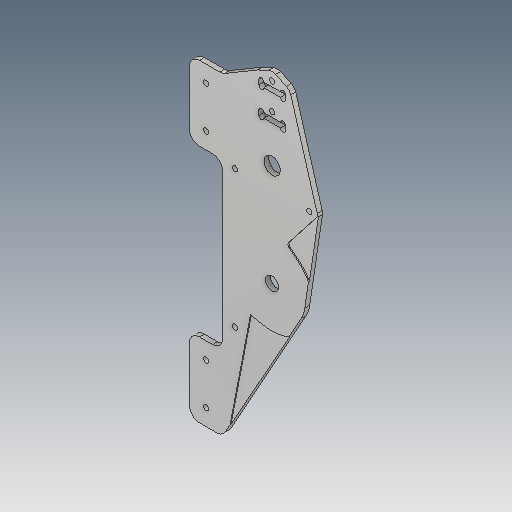
# Autodesk Inventor part: Pitch_B
Saved by Autodesk Inventor 2019.4 (Build 234330000, 330)
## iProperties
Created: 2019-06-11
Part Number: Pitch_B
Material: アルミニウム
Document SubType Name: Modeling
Designer: AzLIer
Density: 2.7 g/cm^3
Appearance: アルミニウム - つや出し
Mass: 74.3393 g
Surface Area: 210.238 cm^2
Volume: 27.5331 cm^3
Author: AzLIer
Autodesk Inventor part; units mm, degrees
ref_plane "YZ Plane" through (0, 0, 0) normal (1, 0, 0) x (0, 1, 0)
ref_plane "XZ Plane" through (0, 0, 0) normal (0, 1, 0) x (-1, 0, 0)
ref_plane "XY Plane" through (0, 0, 0) normal (0, 0, 1) x (1, 0, 0)
sketch "スケッチ1" plane through (0, 0, 0) normal (0, 0, 1) x (1, 0, 0)
  arc A0 (0, -120) -> (0, 120) centre (0, 0) ccw
  line L0 (0, 120) -> (0, -120)
  dimension "d0" = 120
  constraints: 2 end point, 2 point on circle, 1 centre point, 1 coincident, 1 vertical
  measures "d0" radius of A0
extrude "押し出し1" add sketch "スケッチ1" along normal blind 3
sketch "スケッチ2" plane through (0, 0, 0) normal (0, 0, -1) x (-1, 0, 0)
  line L0 (0, 120) -> (0, -120) projected
  line L1 (0, 120) -> (50, 120)
  line L2 (50, 120) -> (50, -120)
  line L3 (50, -120) -> (0, -120)
  line L4 (0, -120) -> (0, 120)
  point P0 (0, 0)
  dimension "d3" = 50
  constraints: 8 end point, 2 parallel, 1 horizontal, 1 perpendicular, 1 point on line
  measures "d3" distance of L0.start L1.end
extrude "押し出し2" add sketch "スケッチ2" against normal blind 3
sketch "スケッチ3" plane through (0, 0, 3) normal (0, 0, 1) x (1, 0, 0)
  line L0 (-50, 120) -> (-50, -120) projected
  line L1 (-50, 40) -> (-40, 40)
  line L2 (-40, 40) -> (-40, -40)
  line L3 (-40, -40) -> (-50, -40)
  line L4 (-50, -40) -> (-50, 40)
  line L5 (-40, 60) -> (-40, -60) construction
  circle A0 centre (-40, 60) radius 1.6
  circle A1 centre (-40, -60) radius 1.6
  point P0 (0, 0)
  point P1 (-50, 0)
  point P2 (-40, 0)
  point P3 (-40, 0)
  dimension "d8" = 10
  dimension "d9" = 80
  dimension "d10" = 120
  dimension "d11" = 10
  dimension "d12" = 3.2
  dimension "d13" = 3.2
  constraints: 10 end point, 4 midpoint, 3 coincident, 2 centre point, 2 parallel, 1 horizontal, 1 perpendicular, 1 vertical
  measures "d8" distance of L2.end L3.end
  measures "d9" distance of L1.end L2.end
  measures "d10" distance of L5.start L5.end
  measures "d11" distance between parallel lines of L0 L5
  measures "d12" diameter of A0
  measures "d13" diameter of A1
extrude "押し出し3" cut sketch "スケッチ3" against normal through all
sketch "スケッチ4" plane through (0, 0, 3) normal (0, 0, 1) x (1, 0, 0)
  circle A0 centre (0, 0) radius 4
  dimension "d14" = 8
  constraints: 1 centre point, 1 coincident
  measures "d14" diameter of A0
extrude "押し出し4" cut sketch "スケッチ4" against normal blind 3
sketch "スケッチ5" plane through (0, 0, 3) normal (0, 0, 1) x (1, 0, 0)
  circle A0 centre (0, 61.8122) radius 3 projected
  circle A1 centre (0, 61.8122) radius 5
  point P0 (0, 0)
  dimension "d17" = 10
  constraints: 1 centre point, 1 coincident
  measures "d17" diameter of A1
extrude "押し出し5" cut sketch "スケッチ5" against normal blind 3 contours A0 | A1
sketch "スケッチ7" plane through (0, 0, 3) normal (0, 0, 1) x (1, 0, 0)
  line L0 (15.7, 89.1122) -> (-15.7, 89.1122) projected
  line L1 (8, 87.1122) -> (-8, 87.1122)
  line L2 (-8, 87.1122) -> (-8, 84.1122)
  line L3 (-8, 84.1122) -> (8, 84.1122)
  line L4 (8, 84.1122) -> (8, 87.1122)
  arc A0 (-8, 84.1122) -> (-5, 84.1122) centre (-6.5, 84.1122) ccw
  arc A1 (5, 84.1122) -> (8, 84.1122) centre (6.5, 84.1122) ccw
  arc A2 (8, 87.1122) -> (5, 87.1122) centre (6.5, 87.1122) ccw
  arc A3 (-5, 87.1122) -> (-8, 87.1122) centre (-6.5, 87.1122) ccw
  circle A4 centre (0, 90.1122) radius 1.6
  point P0 (0, 0)
  point P1 (0, 87.1122)
  point P2 (0, 89.1122)
  dimension "d20" = 2
  dimension "d21" = 16
  dimension "d22" = 3
  dimension "d23" = 1.5
  dimension "d26" = 3.2
  dimension "d27" = 3
  constraints: 8 end point, 8 point on circle, 8 point on line, 5 centre point, 3 equal radius, 2 midpoint, 2 parallel, 2 vertical alignment, 1 horizontal, 1 perpendicular
  measures "d20" distance between parallel lines of L0 L1
  measures "d21" distance of L2.end L3.end
  measures "d22" distance of L3.end L1.start
  measures "d23" radius of A2
  measures "d26" diameter of A4
  measures "d27" distance of point (0, 87.112) A4.centre
extrude "押し出し6" cut sketch "スケッチ7" against normal blind 3
pattern_linear "矩形状パターン1" count 2 spacing 16 along (0, 1, 0) of "押し出し6"
sketch "スケッチ9" plane through (0, 0, 3) normal (0, 0, 1) x (1, 0, 0)
  circle A0 centre (0, 61.8122) radius 4 construction
  circle A1 centre (0, 0) radius 4 construction
  circle A2 centre (22.5, 49) radius 1.6 projected
  circle A3 centre (-22.5, -34) radius 1.6 projected
  circle A4 centre (-22.5, 49) radius 1.6 projected
  line L0 (25.0237, 50.6221) -> (12.6183, 69.9225) construction
  arc A5 (12.6183, 69.9225) -> (-12.6183, 69.9226) centre (0, 61.8122) ccw construction
  line L1 (-12.6183, 69.9226) -> (-25.0237, 50.6221) construction
  arc A6 (-25.0237, 50.6221) -> (-25.5, 49) centre (-22.5, 49) ccw construction
  line L2 (-25.5, 49) -> (-25.5, -34) construction
  arc A7 (-25.5, -34) -> (-20.5963, -36.3186) centre (-22.5, -34) ccw construction
  line L3 (-20.5963, -36.3186) -> (9.5184, -11.5931) construction
  arc A8 (9.5184, -11.5931) -> (14.6828, -3.0686) centre (0, 0) ccw construction
  line L4 (14.6828, -3.0686) -> (25.4366, 48.3863) construction
  arc A9 (25.4366, 48.3863) -> (25.0237, 50.6221) centre (22.5, 49) ccw construction
  point P0 (0, 0)
extrude "押し出し8" cut sketch "スケッチ9" against normal blind 3
sketch "スケッチ8" plane through (0, 0, 3) normal (0, 0, 1) x (1, 0, 0)
  arc A0 (17.4743, -9.7287) -> (19.7797, -2.9601) centre (0, 0) ccw
  line L0 (17.4743, -9.7287) -> (-30, -95)
  circle A1 centre (22.5, 49) radius 1.6 projected
  circle A2 centre (-22.5, 49) radius 1.6 projected
  circle A3 centre (-22.5, -34) radius 1.6 projected
  arc A4 (27.4449, 48.26) -> (27.2948, 50.4177) centre (22.5, 49) ccw
  line L1 (27.4449, 48.26) -> (19.7797, -2.9601)
  arc A5 (11.2948, 104.5299) -> (8.5953, 107.652) centre (6.5, 103.1122) ccw
  arc A6 (2.0953, 110.652) -> (-2.0953, 110.652) centre (0, 106.1122) ccw
  line L2 (8.5953, 107.652) -> (2.0953, 110.652)
  line L3 (27.2948, 50.4177) -> (11.2948, 104.5299)
  line L4 (-2.0953, 110.652) -> (-8.5953, 107.652)
  arc A7 (-8.5953, 107.652) -> (-9.0487, 107.4138) centre (-6.5, 103.1122) ccw
  line L5 (-9.0487, 107.4138) -> (-30, 95)
  circle A8 centre (-40, 85) radius 1.6 projected
  line L6 (-50, 50) -> (-30, 50) projected
  line L7 (-30, 95) -> (-30, 50) projected
  line L8 (-50, 95) -> (-30, 95) projected
  line L9 (-50, 50) -> (-50, 95) projected
  circle A9 centre (-40, 60) radius 1.6 projected
  circle A10 centre (-40, -85) radius 1.6 projected
  circle A11 centre (-40, -60) radius 1.6 projected
  line L10 (-30, -50) -> (-50, -50) projected
  line L11 (-50, -95) -> (-50, -50) projected
  line L12 (-30, -95) -> (-50, -95) projected
  line L13 (-30, -50) -> (-30, -95) projected
  line L14 (-30, 50) -> (-30, -50)
  point P0 (-47, -55)
  point P1 (-50, -80)
  point P2 (-35, 50)
  point P3 (-35, 95)
  point P4 (-35, -50)
  point P5 (-35, -95)
  dimension "d41" = 10
  dimension "d44" = 5
  dimension "d48" = 20
  constraints: 14 end point, 10 point on circle, 10 tangent, 5 centre point, 4 point on line, 3 coincident, 2 equal radius, 1 perpendicular
  measures "d41" diameter of A4
  measures "d44" radius of A5
  measures "d48" radius of A0
extrude "押し出し9" cut sketch "スケッチ8" against normal through all contours L0 L13 L14 L7 L5 A7 L4 A6 L2 A5 L3 A4 L1 A0 | L12 L11 L10 L13 | L6 L9 L8 L7 | A1 | A2 | A3 keep common part
fillet "フィレット2" radius 6 8 edges at (-50, 50, 1.5) (-30, 50, 1.5) (-30, -50, 1.5) (-50, -50, 1.5) (-50, 95, 1.5) (-30, 95, 1.5) (-50, -95, 1.5) (-30, -95, 1.5)
sketch "スケッチ10" plane through (0, 0, 3) normal (0, 0, 1) x (1, 0, 0)
  arc A0 (-33.5268, -95) -> (-28.2845, -91.9186) centre (-33.5268, -89) ccw projected
  line L0 (17.4743, -9.7287) -> (-28.2845, -91.9186) projected
  arc A1 (17.4743, -9.7287) -> (19.7797, -2.9601) centre (0, 0) ccw projected
  line L1 (27.4449, 48.26) -> (19.7797, -2.9601) projected
  arc A2 (27.4449, 48.26) -> (27.2948, 50.4177) centre (22.5, 49) ccw projected
  line L2 (11.2948, 104.5299) -> (27.2948, 50.4177) projected
  arc A3 (11.2948, 104.5299) -> (8.5953, 107.652) centre (6.5, 103.1122) ccw projected
  line L3 (2.0953, 110.652) -> (8.5953, 107.652) projected
  arc A4 (2.0953, 110.652) -> (-2.0953, 110.652) centre (0, 106.1122) ccw projected
  line L4 (-8.5953, 107.652) -> (-2.0953, 110.652) projected
  arc A5 (-8.5953, 107.652) -> (-9.0487, 107.4138) centre (-6.5, 103.1122) ccw projected
  line L5 (-28.5856, 95.8381) -> (-9.0487, 107.4138) projected
  arc A6 (-31.6441, 95) -> (-28.5856, 95.8381) centre (-31.6441, 101) ccw projected
  line L6 (-44, 95) -> (-31.6441, 95) projected
  arc A7 (-44, 95) -> (-50, 89) centre (-44, 89) ccw projected
  line L7 (-50, 89) -> (-50, 56) projected
  arc A8 (-50, 56) -> (-44, 50) centre (-44, 56) ccw projected
  line L8 (-36, 50) -> (-44, 50) projected
  arc A9 (-30, 44) -> (-36, 50) centre (-36, 44) ccw projected
  line L9 (-30, -44) -> (-30, 44) projected
  arc A10 (-36, -50) -> (-30, -44) centre (-36, -44) ccw projected
  line L10 (-44, -50) -> (-36, -50) projected
  arc A11 (-44, -50) -> (-50, -56) centre (-44, -56) ccw projected
  line L11 (-50, -56) -> (-50, -89) projected
  arc A12 (-50, -89) -> (-44, -95) centre (-44, -89) ccw projected
  line L12 (-33.5268, -95) -> (-44, -95) projected
  circle A13 centre (-40, -85) radius 1.6 projected
  circle A14 centre (-40, 85) radius 1.6 projected
  circle A15 centre (-22.5, -34) radius 1.6 projected
  circle A16 centre (22.5, 49) radius 1.6 projected
  circle A17 centre (-22.5, 49) radius 1.6 projected
  circle A18 centre (0, 106.1122) radius 1.6 projected
  arc A19 (8, 103.1122) -> (5, 103.1122) centre (6.5, 103.1122) ccw projected
  line L13 (8, 103.1122) -> (8, 100.1122) projected
  arc A20 (5, 100.1122) -> (8, 100.1122) centre (6.5, 100.1122) ccw projected
  line L14 (5, 100.1122) -> (-5, 100.1122) projected
  arc A21 (-8, 100.1122) -> (-5, 100.1122) centre (-6.5, 100.1122) ccw projected
  line L15 (-8, 100.1122) -> (-8, 103.1122) projected
  arc A22 (-5, 103.1122) -> (-8, 103.1122) centre (-6.5, 103.1122) ccw projected
  line L16 (-5, 103.1122) -> (5, 103.1122) projected
  circle A23 centre (0, 90.1122) radius 1.6 projected
  arc A24 (8, 87.1122) -> (5, 87.1122) centre (6.5, 87.1122) ccw projected
  line L17 (8, 87.1122) -> (8, 84.1122) projected
  arc A25 (5, 84.1122) -> (8, 84.1122) centre (6.5, 84.1122) ccw projected
  line L18 (5, 84.1122) -> (-5, 84.1122) projected
  arc A26 (-8, 84.1122) -> (-5, 84.1122) centre (-6.5, 84.1122) ccw projected
  line L19 (-8, 84.1122) -> (-8, 87.1122) projected
  arc A27 (-5, 87.1122) -> (-8, 87.1122) centre (-6.5, 87.1122) ccw projected
  line L20 (-5, 87.1122) -> (5, 87.1122) projected
  circle A28 centre (0, 61.8122) radius 5 projected
  circle A29 centre (0, 0) radius 4 projected
  circle A30 centre (-40, 60) radius 1.6 projected
  circle A31 centre (-40, -60) radius 1.6 projected
  line L21 (27.4974, 48.8393) -> (9.9725, 26.4915)
  circle A32 centre (66.9129, -143.1316) radius 1.6 projected
  circle A33 centre (14.399, -30.8005) radius 1.6 projected
  circle A34 centre (20.7515, -44.3889) radius 1.6 projected
  circle A35 centre (58.443, -125.0137) radius 1.6 projected
  line L22 (4.2168, -26.7296) -> (17.8052, -20.3771) projected
  line L23 (4.2168, -26.7296) -> (63.5067, -153.555) projected
  line L24 (77.0952, -147.2025) -> (63.5067, -153.555) projected
  line L25 (17.8052, -20.3771) -> (77.0952, -147.2025) projected
  line L26 (15.427, 19.6725) -> (10.3121, 23.6835)
  arc A36 (9.9725, 26.4915) -> (10.3121, 23.6835) centre (11.5463, 25.2573) ccw
  circle A37 centre (-26.1999, -135.4901) radius 1.6 projected
  circle A38 centre (-6.455, -33.3816) radius 1.6 projected
  circle A39 centre (-9.3028, -48.1088) radius 1.6 projected
  circle A40 centre (-23.352, -120.7629) radius 1.6 projected
  line L27 (-12.2998, -24.1032) -> (2.4274, -26.951) projected
  line L28 (-12.2998, -24.1032) -> (-35.0823, -141.9207) projected
  line L29 (-20.3551, -144.7685) -> (-35.0823, -141.9207) projected
  line L30 (2.4274, -26.951) -> (-20.3551, -144.7685) projected
  line L31 (-4.7464, -24.5453) -> (-13.0918, -22.9315)
  line L32 (-13.0918, -22.9315) -> (-25.446, -86.8203)
  arc A41 (-4.7464, -24.5453) -> (10.1778, -22.8345) centre (0, 0) ccw
  arc A42 (21.9998, 11.8747) -> (15.427, 19.6725) centre (0, 0) ccw
  dimension "d54" = 2
  dimension "d55" = 1
  dimension "d56" = 1
  dimension "d57" = 25
  constraints: 8 end point, 7 point on circle, 4 tangent, 3 centre point, 3 point on line, 2 perpendicular, 1 coincident, 1 concentric, 1 parallel, 1 other
  measures "d54" radius of A36
  measures "d56" distance between parallel lines of L28 L32
  measures "d57" radius of A41
extrude "押し出し11" cut sketch "スケッチ10" against normal blind 0.6 contours L32 L31 A41 L0 L22 L23 L30 L27 L28 | L28 L27 L30 L0 | L23 L22 L0 | A42 L26 A36 L21 A2 L1 | A33 | A38 | A39
equation "\"d27\" = d22"
